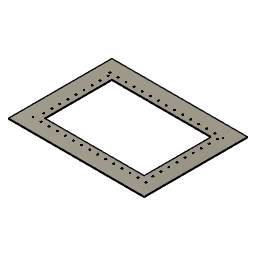
m v1 (Autodesk Fusion 360 design; units mm, degrees)
Autodesk Fusion 360 part; units mm, degrees
sketch "スケッチ1" plane through (0, 0, 0) normal (0, 0, 1) x (1, 0, 0)
  line L0 (-300, -200) -> (300, -200)
  line L1 (300, -200) -> (300, 200)
  line L2 (300, 200) -> (-300, 200)
  line L3 (-300, 200) -> (-300, -200)
  line L4 (-119.9867, 518.3256) -> (720.0133, 518.3256)
  line L5 (720.0133, 518.3256) -> (720.0133, -121.6744)
  line L6 (720.0133, -121.6744) -> (-119.9867, -121.6744)
  line L7 (-119.9867, -121.6744) -> (-119.9867, 518.3256)
  line L8 (-7.9867, 406.3256) -> (608.0133, 406.3256)
  line L9 (608.0133, 406.3256) -> (608.0133, -9.6744)
  line L10 (608.0133, -9.6744) -> (-7.9867, -9.6744)
  line L11 (-7.9867, -9.6744) -> (-7.9867, 406.3256)
  circle A0 centre (-50, -39.6744) radius 5
  circle A1 centre (-37.9867, 13.9976) radius 5
  line L12 (0, -200) -> (0, 200)
  line L13 (-300, 0) -> (300, 0)
  line L14 (300.0133, 518.3256) -> (300.0133, -121.6744)
  line L15 (-119.9867, 198.3256) -> (720.0133, 198.3256)
  circle A2 centre (638.0133, 13.9976) radius 5
  circle A3 centre (-50, 436.3256) radius 5
  circle A4 centre (0, -39.6744) radius 5
  circle A5 centre (0, 436.3256) radius 5
  circle A6 centre (50, -39.6744) radius 5
  circle A7 centre (50, 436.3256) radius 5
  circle A8 centre (100, -39.6744) radius 5
  circle A9 centre (100, 436.3256) radius 5
  circle A10 centre (150, -39.6744) radius 5
  circle A11 centre (150, 436.3256) radius 5
  circle A12 centre (200, -39.6744) radius 5
  circle A13 centre (200, 436.3256) radius 5
  circle A14 centre (250, -39.6744) radius 5
  circle A15 centre (250, 436.3256) radius 5
  circle A16 centre (300, -39.6744) radius 5
  circle A17 centre (300, 436.3256) radius 5
  circle A18 centre (350, -39.6744) radius 5
  circle A19 centre (350, 436.3256) radius 5
  circle A20 centre (400, -39.6744) radius 5
  circle A21 centre (400, 436.3256) radius 5
  circle A22 centre (450, -39.6744) radius 5
  circle A23 centre (450, 436.3256) radius 5
  circle A24 centre (500, -39.6744) radius 5
  circle A25 centre (500, 436.3256) radius 5
  circle A26 centre (550, -39.6744) radius 5
  circle A27 centre (550, 436.3256) radius 5
  circle A28 centre (600, -39.6744) radius 5
  circle A29 centre (600, 436.3256) radius 5
  circle A30 centre (650, -39.6744) radius 5
  circle A31 centre (650, 436.3256) radius 5
  circle A32 centre (-37.9867, 63.9976) radius 5
  circle A33 centre (638.0133, 63.9976) radius 5
  circle A34 centre (-37.9867, 113.9976) radius 5
  circle A35 centre (638.0133, 113.9976) radius 5
  circle A36 centre (-37.9867, 163.9976) radius 5
  circle A37 centre (638.0133, 163.9976) radius 5
  circle A38 centre (-37.9867, 213.9976) radius 5
  circle A39 centre (638.0133, 213.9976) radius 5
  circle A40 centre (-37.9867, 263.9976) radius 5
  circle A41 centre (638.0133, 263.9976) radius 5
  circle A42 centre (-37.9867, 313.9976) radius 5
  circle A43 centre (638.0133, 313.9976) radius 5
  circle A44 centre (-37.9867, 363.9976) radius 5
  circle A45 centre (638.0133, 363.9976) radius 5
  circle A46 centre (-37.9867, 413.9976) radius 5
  circle A47 centre (638.0133, 413.9976) radius 5
  dimension "d1" = 600
  dimension "d2" = 400
  dimension "d3" = 840
  dimension "d4" = 640
  dimension "d5" = 10
  dimension "d6" = 10
  dimension "d10" = 50
  dimension "d11" = 0
  dimension "d12" = 616
  dimension "d13" = 416
  dimension "d14" = 616
  dimension "d15" = 416
  dimension "d16" = 30
  dimension "d17" = 50
  dimension "d18" = 30
  dimension "d21" = -50
  dimension "d22" = 0
  dimension "d23" = 55
  constraint horizontal L0
  constraint vertical L1
  constraint horizontal L2
  constraint vertical L3
  constraint horizontal L4
  constraint vertical L5
  constraint horizontal L6
  constraint vertical L7
  constraint horizontal L8
  constraint vertical L9
  constraint horizontal L10
  constraint vertical L11
  constraint midpoint L0 L12.start
  constraint midpoint L2 L12.end
  constraint midpoint L3 L13.start
  constraint midpoint L1 L13.end
  constraint midpoint L13 origin
  constraint midpoint L4 L14.start
  constraint midpoint L6 L14.end
  constraint midpoint L7 L15.start
  constraint midpoint L5 L15.end
  constraint symmetric A1 L14 A2
  constraint symmetric A0 L15 A3
  measures "d1" distance of L0.start L0.end
  measures "d2" distance of L0.start L2.end
  measures "d3" distance of L4.start L4.end
  measures "d4" distance of L4.start L6.end
  measures "d5" diameter of A0
  measures "d6" diameter of A1
  measures "d12" distance of L8.start L8.end
  measures "d13" distance of L8.start L10.end
  measures "d16" distance of L11 A1.centre
  measures "d17" distance of A0.centre L12
  measures "d18" distance of L10 A0.centre
  measures "d23" distance of A0.centre A1.centre
sketch "スケッチ2" plane through (0, 0, 0) normal (0, 0, 1) x (1, 0, 0)
  line L0 (-420, -320) -> (420, -320)
  line L1 (420, -320) -> (420, 320)
  line L2 (420, 320) -> (-420, 320)
  line L3 (-420, 320) -> (-420, -320)
  line L4 (-308, -208) -> (308, -208)
  line L5 (308, -208) -> (308, 208)
  line L6 (308, 208) -> (-308, 208)
  line L7 (-308, 208) -> (-308, -208)
  circle A0 centre (-350, -238) radius 5
  circle A1 centre (-338, -184.3251) radius 5
  line L8 (-300, 200) -> (300, 200) construction
  line L9 (300, 200) -> (300, -200) construction
  line L10 (300, -200) -> (-300, -200) construction
  line L11 (-300, -200) -> (-300, 200) construction
  line L12 (0, 200) -> (0, -200) construction
  line L13 (-300, 0) -> (300, 0) construction
  circle A2 centre (-350, 238) radius 5
  line L14 (0, -200) -> (0, 200)
  circle A3 centre (338, -184.3251) radius 5
  line L15 (-300, 200) -> (-300, -200)
  circle A4 centre (-338, -134.3251) radius 5
  circle A5 centre (338, -134.3251) radius 5
  circle A6 centre (-338, -84.3251) radius 5
  circle A7 centre (338, -84.3251) radius 5
  circle A8 centre (-338, -34.3251) radius 5
  circle A9 centre (338, -34.3251) radius 5
  circle A10 centre (-338, 15.6749) radius 5
  circle A11 centre (338, 15.6749) radius 5
  circle A12 centre (-338, 65.6749) radius 5
  circle A13 centre (338, 65.6749) radius 5
  circle A14 centre (-338, 115.6749) radius 5
  circle A15 centre (338, 115.6749) radius 5
  circle A16 centre (-338, 165.6749) radius 5
  circle A17 centre (338, 165.6749) radius 5
  circle A18 centre (-338, 215.6749) radius 5
  circle A19 centre (338, 215.6749) radius 5
  circle A20 centre (-300, -238) radius 5
  circle A21 centre (-250, -238) radius 5
  circle A22 centre (-200, -238) radius 5
  circle A23 centre (-150, -238) radius 5
  circle A24 centre (-100, -238) radius 5
  circle A25 centre (-50, -238) radius 5
  circle A26 centre (0, -238) radius 5
  circle A27 centre (50, -238) radius 5
  circle A28 centre (100, -238) radius 5
  circle A29 centre (150, -238) radius 5
  circle A30 centre (200, -238) radius 5
  circle A31 centre (250, -238) radius 5
  circle A32 centre (300, -238) radius 5
  circle A33 centre (350, -238) radius 5
  circle A34 centre (-300, 238) radius 5
  circle A35 centre (-250, 238) radius 5
  circle A36 centre (-200, 238) radius 5
  circle A37 centre (-150, 238) radius 5
  circle A38 centre (-100, 238) radius 5
  circle A39 centre (-50, 238) radius 5
  circle A40 centre (0, 238) radius 5
  circle A41 centre (50, 238) radius 5
  circle A42 centre (100, 238) radius 5
  circle A43 centre (150, 238) radius 5
  circle A44 centre (200, 238) radius 5
  circle A45 centre (250, 238) radius 5
  circle A46 centre (300, 238) radius 5
  circle A47 centre (350, 238) radius 5
  line L16 (-300, 0) -> (300, 0)
  dimension "d24" = 840
  dimension "d25" = 640
  dimension "d26" = 616
  dimension "d27" = 416
  dimension "d28" = 10
  dimension "d30" = 10
  dimension "d32" = 600
  dimension "d33" = 400
  dimension "d34" = 308
  dimension "d35" = 208
  dimension "d36" = 30
  dimension "d38" = 30
  dimension "d39" = 55
  dimension "d42" = 50
  dimension "d43" = 0
  dimension "d44" = 50
  dimension "d47" = 0
  dimension "d48" = 50
  dimension "d49" = 420
  dimension "d50" = 320
  constraint horizontal L0
  constraint vertical L1
  constraint horizontal L2
  constraint vertical L3
  constraint horizontal L4
  constraint vertical L5
  constraint horizontal L6
  constraint vertical L7
  constraint horizontal L8
  constraint vertical L9
  constraint horizontal L10
  constraint vertical L11
  constraint midpoint L8 L12.start
  constraint midpoint L10 L12.end
  constraint midpoint L11 L13.start
  constraint midpoint L9 L13.end
  constraint midpoint L13 origin
  constraint symmetric A0 L13 A2
  constraint symmetric A1 L14 A3
  measures "d24" distance of L0.start L0.end
  measures "d25" distance of L0.start L2.end
  measures "d26" distance of L4.start L4.end
  measures "d27" distance of L4.start L6.end
  measures "d28" diameter of A0
  measures "d30" diameter of A1
  measures "d32" distance of L8.start L8.end
  measures "d33" distance of L8.start L10.end
  measures "d34" distance of L7 L12
  measures "d35" distance of L6 L13
  measures "d36" distance of L7 A1.centre
  measures "d38" distance of L4 A0.centre
  measures "d39" distance of A0.centre A1.centre
  measures "d44" distance of A0.centre L15
  measures "d49" distance of L3 origin
  measures "d50" distance of L2 L16
extrude "押し出し1" add sketch "スケッチ2" along normal blind 5
equation "d34 = ( 616 / 2 ) * 1 mm"
equation "d35 = ( 416 / 2 ) * 1 mm"
